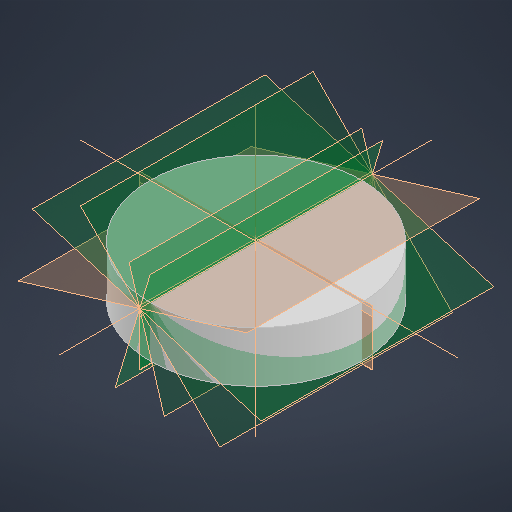
# Autodesk Inventor part: 1in_5mm_mir
Saved by Autodesk Inventor 2026 (Build 300175050, 175E)
## iProperties
Created: 2019-05-24
Part Number: 1in_5mm_mir
Material: Generic
Document SubType Name: Modeling
Designer: Julian
Density: 1 g/cm^3
Appearance: Default
Author: Julian
Autodesk Inventor part; units mm, degrees
ref_plane "YZ Plane" through (0, 0, 0) normal (1, 0, 0) x (0, 1, 0)
ref_plane "XZ Plane" through (0, 0, 0) normal (0, 1, 0) x (-1, 0, 0)
ref_plane "XY Plane" through (0, 0, 0) normal (0, 0, 1) x (1, 0, 0)
sketch "Sketch1" plane through (0, 0, 0) normal (0, 1, 0) x (-1, 0, 0)
  circle A0 centre (0, 0) radius 12.7
  point P0 (-12.7, 0)
  point P1 (0, -12.7)
  dimension "d0" = 25.4
  constraints: 2 coincident, 2 point on circle, 1 centre point
  measures "d0" diameter of A0
extrude "Extrusion1" add sketch "Sketch1" along normal blind 6.096
ref_plane "Work Plane11" through (0, 0, 0) normal (-1, 0, 0) x (0, -1, 0)
ref_plane "Work Plane12" through (0, 0, 0) normal (0, 0, 1) x (0, -1, 0)
ref_plane "Work Plane13" through (0, 6.096, 0) normal (-0.7071, 0.7071, 0) x (0, 0, 1)
ref_plane "Work Plane14" through (0, 6.096, 0) normal (-0.7071, -0.7071, 0) x (0, 0, 1)
ref_plane "Work Plane15" through (0, 0, 0) normal (0, 0, 1) x (0, -1, 0)
ref_plane "Work Plane16" through (0, 0, 0) normal (-1, 0, 0) x (0, -1, 0)
ref_plane "Work Plane20" through (0, 6.096, 0) normal (0, -0.7071, 0.7071) x (1, 0, 0)
ref_plane "Arbeitsebene21" through (0, 0, 0) normal (-0.7071, 0, 0.7071) x (0, -1, 0)
ref_plane "Work Plane23" through (0, 6.096, 0) normal (-0.9239, 0.3827, 0) x (0, 0, -1)
ref_plane "Work Plane22" through (0, 6.096, 0) normal (-0.9239, -0.3827, 0) x (0, 0, 1)
ref_plane "Work Plane30" through (0, 6.096, 0) normal (-0.9808, 0.1951, 0) x (0, 0, -1)
ref_plane "Work Plane31" through (0, 6.096, 0) normal (-0.9808, -0.1951, 0) x (0, 0, 1)
ref_plane "Work Plane32" through (0, 6.096, 0) normal (-0.9569, 0.2903, 0) x (0, 0, -1)
ref_plane "Work Plane33" through (0, 6.096, 0) normal (-0.9569, -0.2903, 0) x (0, 0, 1)
ref_plane "Work Plane36" through (0, 6.096, 0) normal (-0.3827, -0.9239, 0) x (0, 0, 1)
ref_plane "Work Plane38" through (0, 6.096, 0) normal (-0.2903, -0.9569, 0) x (0, 0, -1)
ref_plane "Work Plane37" through (0, 6.096, 0) normal (-0.1951, -0.9808, 0) x (0, 0, 1)
ref_plane "Work Plane39" through (0, 6.096, 0) normal (-0.3827, 0.9239, 0) x (0, 0, -1)
ref_plane "Work Plane41" through (0, 6.096, 0) normal (-0.2903, 0.9569, 0) x (0, 0, 1)
ref_plane "Work Plane40" through (0, 6.096, 0) normal (-0.1951, 0.9808, 0) x (0, 0, -1)
body "Solid1"
